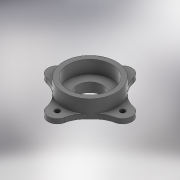
# Autodesk Inventor part: ThrustBearingMount
Saved by Autodesk Inventor 2020.3 (Build 243373000, 373)
## iProperties
Created: 2021-08-03
Part Number: ThrustBearingMount
Material: ABS Plastic
Document SubType Name: Modeling
Designer: justi
Density: 1.06 g/cm^3
Appearance: Smooth - Black
Author: justi
Autodesk Inventor part; units mm, degrees
ref_plane "YZ Plane" through (0, 0, 0) normal (1, 0, 0) x (0, 1, 0)
ref_plane "XZ Plane" through (0, 0, 0) normal (0, 1, 0) x (-1, 0, 0)
ref_plane "XY Plane" through (0, 0, 0) normal (0, 0, 1) x (1, 0, 0)
sketch "Sketch1" plane through (0, 0, 0) normal (1, 0, 0) x (0, 1, 0)
  line L0 (0, 0) -> (0, 23.5) construction
  line L1 (0, 23.5) -> (14, 23.5) construction
  line L2 (14, 23.5) -> (14, 0) construction
  line L3 (14, 23.5) -> (14, 28.5)
  line L4 (14, 28.5) -> (-5, 28.5)
  line L5 (14, 23.5) -> (0, 23.5)
  line L6 (-5, 28.5) -> (-5, 17.5)
  line L7 (-5, 17.5) -> (-10, 17.5)
  line L8 (-14.8, 0) -> (18.8, 0) projected
  line L9 (-10, 0) -> (-10, 13.5) construction
  line L10 (-10, 13.5) -> (0, 13.5)
  line L11 (0, 23.5) -> (0, 13.5)
  line L12 (-10, 17.5) -> (-10, 13.5)
  dimension "d0" = 23.5
  dimension "d1" = 14
  dimension "d2" = 5
  dimension "d3" = 19
  dimension "d8" = 11
  dimension "d9" = 5
  dimension "d11" = 13.5
  constraints: 24 end point, 7 perpendicular, 3 vertical, 2 point on line, 1 collinear, 1 parallel
  measures "d0" distance of L0.start L0.end
  measures "d1" distance of L0.end L1.end
  measures "d2" distance of L1.end L3.end
  measures "d3" distance of L3.end L4.end
  measures "d8" distance of L4.end L6.end
  measures "d9" distance of L6.end L7.end
  measures "d11" distance of L9.start L9.end
revolve "Revolution1" add sketch "Sketch1" angle 360 about axis through (0, -10, 0) along (0, 1, 0)
sketch "Sketch2" plane through (0, -5, 0) normal (0, -1, 0) x (1, 0, 0)
  line L0 (-35, 0) -> (35, 0) construction
  arc A0 (-35, 10) -> (-35, -10) centre (-35, 0) ccw
  arc A1 (35, -10) -> (35, 10) centre (35, 0) ccw
  line L1 (0, -35) -> (0, 35) construction
  arc A2 (-10, -35) -> (10, -35) centre (0, -35) ccw
  arc A3 (10, 35) -> (-10, 35) centre (0, 35) ccw
  line L2 (-10, 35) -> (-10, 10)
  line L3 (-10, -10) -> (-10, -35)
  line L4 (35, 10) -> (10, 10)
  line L5 (-10, 10) -> (-35, 10)
  line L6 (10, -35) -> (10, -10)
  line L7 (10, 10) -> (10, 35)
  line L8 (-35, -10) -> (-10, -10)
  line L9 (10, -10) -> (35, -10)
  circle A4 centre (0, 0) radius 13.5
  dimension "d12" = 35
  dimension "d13" = 20
  dimension "d14" = 35
  dimension "d15" = 20
  constraints: 24 end point, 16 tangent, 8 parallel, 8 point on circle, 5 centre point, 5 coincident, 2 midpoint, 1 horizontal, 1 perpendicular
  measures "d12" distance of point (0, 0) L0.end
  measures "d13" diameter of A1
  measures "d14" distance of point (0, 0) L1.end
  measures "d15" diameter of A3
extrude "Extrusion1" add sketch "Sketch2" against normal blind 5
fillet "Fillet1" radius 27 8 edges at (10, -2.5, 26.688) (26.688, -2.5, 10) (-10, -2.5, 26.688) (-26.688, -2.5, 10) (-26.688, -2.5, -10) (-10, -2.5, -26.688) (10, -2.5, -26.688) (26.688, -2.5, -10)
hole "Hole1" at (0, -5, 35) at (35, -5, 0) at (0, -5, -35) at (-35, -5, 0) direction (0, 1, 0) diameter 5.5 end through all clearance for "Hex Head Bolt" size "M5" standard "Ansi Metric M Profile"
body "Solid1"
